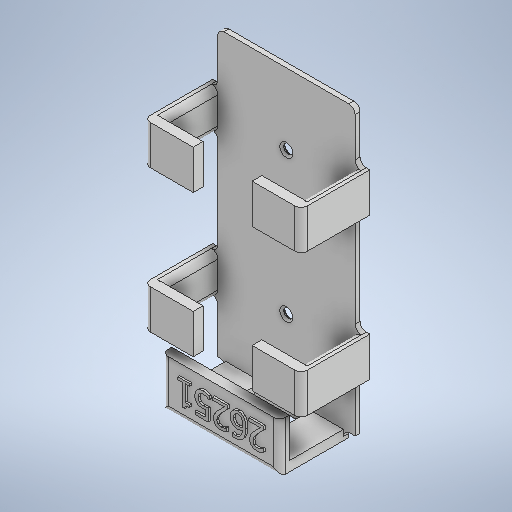
# Autodesk Inventor part: ChonkyPowerBankHolder
Saved by Autodesk Inventor 2025 (Build 290162010, 162A)
## iProperties
Created: 2024-11-16
Part Number: ChonkyPowerBankHolder
Material: Generic
Document SubType Name: Modeling
Designer: ishaa
Density: 1 g/cm^3
Appearance: Default
Author: ishaa
## iProperties of the stored document ChonkyPowerBankHolder_3DPrint.ipt
Created: 2024-12-01
Part Number: ChonkyPowerBankHolder_3DPrint
Material: Generic
Document SubType Name: Modeling
Designer: dcfam
Density: 1 g/cm^3
Appearance: Default
Author: dcfam
Autodesk Inventor part; units mm, degrees
ref_plane "YZ Plane" through (0, 0, 0) normal (1, 0, 0) x (0, 1, 0)
ref_plane "XZ Plane" through (0, 0, 0) normal (0, 1, 0) x (-1, 0, 0)
ref_plane "XY Plane" through (0, 0, 0) normal (0, 0, 1) x (1, 0, 0)
sketch "Sketch1" plane through (0, 0, 0) normal (0, 0, 1) x (1, 0, 0)
  line L0 (-35, -72.5) -> (35, -72.5)
  line L1 (35, -72.5) -> (35, 72.5)
  line L2 (35, 72.5) -> (-35, 72.5)
  line L3 (-35, 72.5) -> (-35, -72.5)
  line L4 (-35, -72.5) -> (35, 72.5) construction
  line L5 (35, -72.5) -> (-35, 72.5) construction
  point P0 (0, 0)
  dimension "d0" = 70
  dimension "d1" = 145
  constraints: 12 end point, 2 midpoint, 2 parallel, 1 horizontal, 1 perpendicular
  measures "d0" distance of L2.end L1.end
  measures "d1" distance of L1.end L0.end
extrude "Extrusion1" add sketch "Sketch1" along normal blind 2.5
sketch "Sketch2" plane through (0, 0, 0) normal (0, 0, -1) x (-1, 0, 0)
  line L0 (-35, 72.5) -> (35, 72.5) construction
  line L1 (0, 72.5) -> (0, -72.5) construction
  line L2 (35, -72.5) -> (-35, -72.5) construction
  line L3 (35, 0) -> (-35, 0) construction
  line L4 (-35, -72.5) -> (-35, 72.5) construction
  line L5 (-35, 0) -> (-35, -72.5) construction
  line L6 (-35, -36.25) -> (35, -36.25) construction
  line L7 (35, 72.5) -> (35, -72.5) construction
  line L8 (-35, -72.5) -> (-35, 72.5) construction
  line L9 (-35, 72.5) -> (35, 72.5) construction
  line L10 (35, 72.5) -> (35, -72.5) construction
  line L11 (35, -72.5) -> (-35, -72.5) construction
  line L12 (-35, 72.5) -> (-35, 0) construction
  line L13 (-35, 36.25) -> (35, 36.25) construction
  line L14 (-35, 46.25) -> (-40, 46.25)
  line L15 (-40, 46.25) -> (-40, 26.25)
  line L16 (-40, 26.25) -> (-35, 26.25)
  line L17 (-35, 26.25) -> (-35, 46.25)
  line L18 (-35, 36.25) -> (-23.1595, 36.25) construction
  line L19 (35, 46.25) -> (40, 46.25)
  line L20 (40, 46.25) -> (40, 26.25)
  line L21 (40, 26.25) -> (35, 26.25)
  line L22 (35, 26.25) -> (35, 46.25)
  line L23 (-35, -46.25) -> (-40, -46.25)
  line L24 (-40, -46.25) -> (-40, -26.25)
  line L25 (-40, -26.25) -> (-35, -26.25)
  line L26 (-35, -26.25) -> (-35, -46.25)
  line L27 (40, -26.25) -> (35, -26.25)
  line L28 (40, -46.25) -> (40, -26.25)
  line L29 (35, -46.25) -> (40, -46.25)
  line L30 (35, -26.25) -> (35, -46.25)
  line L31 (-29.0797, -72.5) -> (30.9203, -72.5)
  line L32 (30.9203, -72.5) -> (30.9203, -77.5)
  line L33 (30.9203, -77.5) -> (-29.0797, -77.5)
  line L34 (-29.0797, -77.5) -> (-29.0797, -72.5)
  point P0 (0, 0)
  dimension "d4" = 5
  dimension "d5" = 20
  dimension "d6" = 60
  dimension "d7" = 5
  constraints: 54 end point, 12 symmetric about line, 6 midpoint, 4 parallel, 4 perpendicular, 4 point on line, 3 collinear, 3 horizontal
  measures "d4" distance of L16.end L15.end
  measures "d5" distance of L15.end L14.end
  measures "d6" distance of L32.end L33.end
  measures "d7" distance of L31.end L32.end
extrude "Extrusion2" add sketch "Sketch2" against normal blind 35
sketch "Sketch3" plane through (-30.9203, -72.5, 2.5) normal (0, 1, 0) x (1, 0, 0)
  line L0 (0, 0) -> (60, 0) projected
  line L1 (0, 0) -> (0, -32.5) projected
  line L2 (60, -32.5) -> (0, -32.5) projected
  line L3 (60, 0) -> (60, -32.5) projected
  line L4 (60, -32.5) -> (0, -32.5)
  line L5 (0, -32.5) -> (0, -27.5)
  line L6 (0, -27.5) -> (60, -27.5)
  line L7 (60, -27.5) -> (60, -32.5)
  point P0 (30.9203, 2.5)
  dimension "d10" = 5
  constraints: 8 end point, 2 parallel, 1 horizontal, 1 perpendicular, 1 point on line
  measures "d10" distance of L4.end L5.end
sketch "Sketch4" plane through (35, 26.25, 2.5) normal (-1, 0, 0) x (0, 0, 1)
  line L0 (0, 0) -> (0, 20) projected
  line L1 (0, 0) -> (32.5, 0) projected
  line L2 (32.5, 20) -> (32.5, 0) projected
  line L3 (0, 20) -> (32.5, 20) projected
  line L4 (0, -72.5) -> (0, -52.5) projected
  line L5 (0, -72.5) -> (32.5, -72.5) projected
  line L6 (32.5, -52.5) -> (32.5, -72.5) projected
  line L7 (0, -52.5) -> (32.5, -52.5) projected
  line L8 (32.5, 20) -> (27.5, 20)
  line L9 (27.5, 20) -> (27.5, 0)
  line L10 (27.5, 0) -> (32.5, 0)
  line L11 (32.5, 0) -> (32.5, 20)
  line L12 (0, -52.5) -> (0, 0) projected
  line L13 (0, -26.25) -> (53.9685, -26.25) construction
  line L14 (0, -52.5) -> (32.5, -52.5)
  line L15 (32.5, -72.5) -> (32.5, -52.5)
  line L16 (0, -72.5) -> (32.5, -72.5)
  line L17 (27.5, -72.5) -> (27.5, -52.5)
  point P0 (-2.5, -26.25)
  dimension "d11" = 5
  constraints: 18 end point, 3 symmetric about line, 2 horizontal, 2 parallel, 2 point on line, 1 midpoint, 1 perpendicular
  measures "d11" distance of L10.end L9.end
sketch "Sketch5" plane through (-35, -46.25, 2.5) normal (1, 0, 0) x (0, 0, -1)
  line L0 (0, 0) -> (-32.5, 0) projected
  line L1 (2.5, 20) -> (-32.5, 20) projected
  line L2 (-32.5, 0) -> (-27.5, 0)
  line L3 (-27.5, 0) -> (-27.5, 20)
  line L4 (-27.5, 20) -> (-32.5, 20)
  line L5 (-32.5, 20) -> (-32.5, 0)
  line L6 (0, 72.5) -> (0, 20) construction
  line L7 (0, 46.25) -> (-51.5825, 46.25) construction
  line L8 (-32.5, 92.5) -> (-27.5, 92.5)
  line L9 (-27.5, 92.5) -> (-27.5, 72.5)
  line L10 (-27.5, 72.5) -> (-32.5, 72.5)
  line L11 (-32.5, 72.5) -> (-32.5, 92.5)
  point P0 (2.5, 46.25)
  dimension "d12" = 5
  constraints: 18 end point, 4 symmetric about line, 2 horizontal, 2 parallel, 1 midpoint, 1 perpendicular, 1 point on line
  measures "d12" distance of L4.end L3.end
extrude "Extrusion3" add sketch "Sketch3" along normal blind 20 contours L6 L3 L2 L1
extrude "Extrusion4" add sketch "Sketch5" along normal blind 20
extrude "Extrusion5" add sketch "Sketch4" along normal blind 20 contours L9 L3 L2 L1 | L17 L7 L6 L5
sketch "Sketch6" plane through (0, 0, 2.5) normal (0, 0, 1) x (1, 0, 0)
  line L0 (-30.9203, -77.5) -> (29.0797, -77.5) construction
  line L1 (0, -77.5) -> (0, 72.5) construction
  line L2 (35, 72.5) -> (-35, 72.5) construction
  line L3 (-40, -26.25) -> (-40, -46.25) construction
  line L4 (-40, -46.25) -> (-15, -46.25) construction
  line L5 (-15, -26.25) -> (-15, -46.25) construction
  line L6 (-40, -26.25) -> (-15, -26.25) construction
  line L7 (-15, -26.25) -> (-15, -46.25) construction
  line L8 (-15, -36.25) -> (15, -36.25) construction
  line L9 (15, -46.25) -> (15, -26.25) construction
  circle A0 centre (0, -36.25) radius 2.35
  line L10 (-35, 26.25) -> (-35, -26.25) construction
  line L11 (-35, 0) -> (35, 0) construction
  circle A1 centre (0, 36.25) radius 2.35
  point P0 (0, 0)
  dimension "d19" = 4.7
  constraints: 6 end point, 5 midpoint, 2 centre point, 1 horizontal, 1 point on line, 1 symmetric about line, 1 other
  measures "d19" diameter of A0
extrude "Extrusion6" cut sketch "Sketch6" against normal blind 20
chamfer "Chamfer1" distance 1 angle 45 4 edges at (-2.35, -36.25, 2.5) (-2.35, 36.25, 2.5) (-2.35, -36.25, 0) (-2.35, 36.25, 0)
fillet "Fillet1" radius 3.175 10 edges at (35, -46.25, 1.25) (35, -26.25, 1.25) (35, 46.25, 1.25) (35, 26.25, 1.25) (29.0797, -72.5, 1.25) (-30.9203, -72.5, 1.25) (-35, -46.25, 1.25) (-35, -26.25, 1.25) (-35, 26.25, 1.25) (-35, 46.25, 1.25)
fillet "Fillet2" radius 3.175 2 edges at (-35, 72.5, 1.25) (35, 72.5, 1.25)
fillet "Fillet3" radius 3.175 4 edges at (-40, -36.25, 35) (-40, 36.25, 35) (40, -36.25, 35) (40, 36.25, 35)
fillet "Fillet4" radius 3.175 3 edges at (-0.9203, -77.5, 35) (-30.9203, -65, 35) (29.0797, -65, 35)
fillet "Fillet5" radius 3.175 8 edges at (-35, 46.25, 16.25) (35, 46.25, 16.25) (-35, -26.25, 16.25) (35, -26.25, 16.25) (-35, 26.25, 16.25) (35, 26.25, 16.25) (35, -46.25, 16.25) (-35, -46.25, 16.25)
sketch "Sketch7" plane through (0, 0, 35) normal (0, 0, 1) x (1, 0, 0)
  line L0 (22.7543, -70.5434) -> (-153.14, -70.5434) construction
  line L1 (-153.14, -70.5434) -> (-153.14, -5.5157) construction
  line L2 (-153.14, -5.5157) -> (22.7543, -5.5157) construction
  line L3 (22.7543, -5.5157) -> (22.7543, -70.5434) construction
  line L4 (14.303, -58.0303) -> (21.8606, -58.0303)
  line L5 (21.8606, -58.0303) -> (21.8606, -59.7682)
  spline S0 degree 2 poles (21.8606, -59.7682) (21.0462, -60.5329) (19.5963, -61.953) (18.9011, -62.7177) knots 0 0 0 1 2 2 2
  spline S1 degree 2 poles (18.9011, -62.7177) (17.5008, -64.257) (16.4779, -66.1042) (16.4779, -67.0874) knots 0 0 0 1 2 2 2
  spline S2 degree 2 poles (16.4779, -67.0874) (16.4779, -67.6038) (16.7957, -68.3784) (17.0837, -68.6267) knots 0 0 0 1 2 2 2
  spline S3 degree 2 poles (17.0837, -68.6267) (17.3717, -68.875) (18.1265, -69.1232) (18.5833, -69.1232) knots 0 0 0 1 2 2 2
  spline S4 degree 2 poles (18.5833, -69.1232) (19.0203, -69.1232) (19.9141, -68.9047) (20.3212, -68.7359) knots 0 0 0 1 2 2 2
  spline S5 degree 2 poles (20.3212, -68.7359) (20.6688, -68.5969) (21.3143, -68.1996) (21.513, -68.0606) knots 0 0 0 1 2 2 2
  line L6 (21.513, -68.0606) -> (21.6023, -68.0606)
  line L7 (21.6023, -68.0606) -> (21.6023, -69.8085)
  spline S6 degree 2 poles (21.6023, -69.8085) (21.0959, -70.0567) (19.2785, -70.5434) (18.4641, -70.5434) knots 0 0 0 1 2 2 2
  spline S7 degree 2 poles (18.4641, -70.5434) (16.7461, -70.5434) (14.8095, -68.726) (14.8095, -67.1767) knots 0 0 0 1 2 2 2
  spline S8 degree 2 poles (14.8095, -67.1767) (14.8095, -66.4518) (15.1472, -65.2402) (15.4451, -64.7238) knots 0 0 0 1 2 2 2
  spline S9 degree 2 poles (15.4451, -64.7238) (15.743, -64.1875) (16.607, -63.1348) (17.0837, -62.6283) knots 0 0 0 1 2 2 2
  spline S10 degree 2 poles (17.0837, -62.6283) (17.8583, -61.7842) (19.7552, -59.9768) (20.3212, -59.4504) knots 0 0 0 1 2 2 2
  line L8 (20.3212, -59.4504) -> (14.303, -59.4504)
  line L9 (14.303, -59.4504) -> (14.303, -58.0303)
  spline S11 degree 2 poles (4.9182, -62.0027) (4.9182, -61.0592) (5.5439, -59.4603) (6.0702, -58.9241) knots 0 0 0 1 2 2 2
  spline S12 degree 2 poles (6.0702, -58.9241) (6.6164, -58.358) (7.9869, -57.7721) (8.8112, -57.7721) knots 0 0 0 1 2 2 2
  spline S13 degree 2 poles (8.8112, -57.7721) (9.6355, -57.7721) (10.996, -58.3282) (11.5124, -58.8843) knots 0 0 0 1 2 2 2
  spline S14 degree 2 poles (11.5124, -58.8843) (12.148, -59.5497) (12.863, -61.7842) (12.863, -63.4129) knots 0 0 0 1 2 2 2
  spline S15 degree 2 poles (12.863, -63.4129) (12.863, -65.0118) (12.2076, -67.5839) (11.5223, -68.5373) knots 0 0 0 1 2 2 2
  spline S16 degree 2 poles (11.5223, -68.5373) (10.857, -69.4708) (8.7516, -70.5136) (7.3712, -70.5136) knots 0 0 0 1 2 2 2
  spline S17 degree 2 poles (7.3712, -70.5136) (6.964, -70.5136) (6.249, -70.4341) (5.9808, -70.3447) knots 0 0 0 1 2 2 2
  line L10 (5.9808, -70.3447) -> (5.9808, -68.7657)
  line L11 (5.9808, -68.7657) -> (6.0504, -68.7657)
  spline S18 degree 2 poles (6.0504, -68.7657) (6.2788, -68.8849) (7.113, -69.0934) (7.5897, -69.0934) knots 0 0 0 1 2 2 2
  spline S19 degree 2 poles (7.5897, -69.0934) (9.119, -69.0934) (10.996, -67.0278) (11.1748, -65.0019) knots 0 0 0 1 2 2 2
  spline S20 degree 2 poles (11.1748, -65.0019) (10.5888, -65.409) (9.3574, -65.8559) (8.6225, -65.8559) knots 0 0 0 1 2 2 2
  spline S21 degree 2 poles (8.6225, -65.8559) (7.9075, -65.8559) (6.8349, -65.5679) (6.249, -65.131) knots 0 0 0 1 2 2 2
  spline S22 degree 2 poles (6.249, -65.131) (5.5737, -64.6245) (4.9182, -63.0554) (4.9182, -62.0027) knots 0 0 0 1 2 2 2
  spline S23 degree 2 poles (6.5866, -61.9332) (6.5866, -62.6879) (6.9839, -63.7108) (7.4208, -64.0683) knots 0 0 0 1 2 2 2
  spline S24 degree 2 poles (7.4208, -64.0683) (7.7486, -64.3265) (8.5629, -64.4954) (8.9899, -64.4954) knots 0 0 0 1 2 2 2
  spline S25 degree 2 poles (8.9899, -64.4954) (9.5659, -64.4954) (10.6484, -64.1478) (11.1748, -63.8201) knots 0 0 0 1 2 2 2
  spline S26 degree 2 poles (11.1748, -63.8201) (11.1847, -63.6413) (11.2046, -63.3036) (11.2046, -63.0454) knots 0 0 0 1 2 2 2
  spline S27 degree 2 poles (11.2046, -63.0454) (11.2046, -61.7743) (10.708, -60.2151) (10.3306, -59.8079) knots 0 0 0 1 2 2 2
  spline S28 degree 2 poles (10.3306, -59.8079) (9.983, -59.4206) (9.2283, -59.1128) (8.8012, -59.1128) knots 0 0 0 1 2 2 2
  spline S29 degree 2 poles (8.8012, -59.1128) (7.8081, -59.1128) (6.5866, -60.523) (6.5866, -61.9332) knots 0 0 0 1 2 2 2
  line L12 (-4.0892, -58.0303) -> (3.4683, -58.0303)
  line L13 (3.4683, -58.0303) -> (3.4683, -59.7682)
  spline S30 degree 2 poles (3.4683, -59.7682) (2.6539, -60.5329) (1.204, -61.953) (0.5088, -62.7177) knots 0 0 0 1 2 2 2
  spline S31 degree 2 poles (0.5088, -62.7177) (-0.8914, -64.257) (-1.9143, -66.1042) (-1.9143, -67.0874) knots 0 0 0 1 2 2 2
  spline S32 degree 2 poles (-1.9143, -67.0874) (-1.9143, -67.6038) (-1.5965, -68.3784) (-1.3085, -68.6267) knots 0 0 0 1 2 2 2
  spline S33 degree 2 poles (-1.3085, -68.6267) (-1.0205, -68.875) (-0.2658, -69.1232) (0.191, -69.1232) knots 0 0 0 1 2 2 2
  spline S34 degree 2 poles (0.191, -69.1232) (0.628, -69.1232) (1.5218, -68.9047) (1.929, -68.7359) knots 0 0 0 1 2 2 2
  spline S35 degree 2 poles (1.929, -68.7359) (2.2766, -68.5969) (2.9221, -68.1996) (3.1207, -68.0606) knots 0 0 0 1 2 2 2
  line L14 (3.1207, -68.0606) -> (3.2101, -68.0606)
  line L15 (3.2101, -68.0606) -> (3.2101, -69.8085)
  spline S36 degree 2 poles (3.2101, -69.8085) (2.7036, -70.0567) (0.8862, -70.5434) (0.0719, -70.5434) knots 0 0 0 1 2 2 2
  spline S37 degree 2 poles (0.0719, -70.5434) (-1.6462, -70.5434) (-3.5827, -68.726) (-3.5827, -67.1767) knots 0 0 0 1 2 2 2
  spline S38 degree 2 poles (-3.5827, -67.1767) (-3.5827, -66.4518) (-3.2451, -65.2402) (-2.9472, -64.7238) knots 0 0 0 1 2 2 2
  spline S39 degree 2 poles (-2.9472, -64.7238) (-2.6492, -64.1875) (-1.7852, -63.1348) (-1.3085, -62.6283) knots 0 0 0 1 2 2 2
  spline S40 degree 2 poles (-1.3085, -62.6283) (-0.5339, -61.7842) (1.3629, -59.9768) (1.929, -59.4504) knots 0 0 0 1 2 2 2
  line L16 (1.929, -59.4504) -> (-4.0892, -59.4504)
  line L17 (-4.0892, -59.4504) -> (-4.0892, -58.0303)
  spline S41 degree 2 poles (-13.1563, -61.9232) (-13.1563, -61.0394) (-12.5902, -59.5299) (-12.0738, -58.9737) knots 0 0 0 1 2 2 2
  spline S42 degree 2 poles (-12.0738, -58.9737) (-11.5574, -58.4176) (-10.0181, -57.7721) (-9.0647, -57.7721) knots 0 0 0 1 2 2 2
  spline S43 degree 2 poles (-9.0647, -57.7721) (-8.1907, -57.7721) (-6.4826, -58.1594) (-5.857, -58.4672) knots 0 0 0 1 2 2 2
  line L18 (-5.857, -58.4672) -> (-5.857, -60.2052)
  line L19 (-5.857, -60.2052) -> (-5.9761, -60.2052)
  spline S44 degree 2 poles (-5.9761, -60.2052) (-6.1648, -60.0661) (-6.8699, -59.7086) (-7.297, -59.5497) knots 0 0 0 1 2 2 2
  spline S45 degree 2 poles (-7.297, -59.5497) (-7.7836, -59.3809) (-8.588, -59.1922) (-9.0945, -59.1922) knots 0 0 0 1 2 2 2
  spline S46 degree 2 poles (-9.0945, -59.1922) (-9.591, -59.1922) (-10.5245, -59.5497) (-10.8622, -59.937) knots 0 0 0 1 2 2 2
  spline S47 degree 2 poles (-10.8622, -59.937) (-11.1701, -60.3045) (-11.4878, -61.2777) (-11.4878, -61.9332) knots 0 0 0 1 2 2 2
  spline S48 degree 2 poles (-11.4878, -61.9332) (-11.4878, -62.5886) (-11.1303, -63.4228) (-10.7927, -63.7009) knots 0 0 0 1 2 2 2
  spline S49 degree 2 poles (-10.7927, -63.7009) (-10.4451, -64.0087) (-9.4123, -64.267) (-8.7866, -64.267) knots 0 0 0 1 2 2 2
  spline S50 degree 2 poles (-8.7866, -64.267) (-8.1113, -64.267) (-6.7706, -64.0584) (-6.3634, -63.969) knots 0 0 0 1 2 2 2
  line L20 (-6.3634, -63.969) -> (-6.3634, -70.2852)
  line L21 (-6.3634, -70.2852) -> (-13.0867, -70.2852)
  line L22 (-13.0867, -70.2852) -> (-13.0867, -68.8452)
  line L23 (-13.0867, -68.8452) -> (-7.9425, -68.8452)
  line L24 (-7.9425, -68.8452) -> (-7.9425, -65.5779)
  spline S51 degree 2 poles (-7.9425, -65.5779) (-8.2404, -65.6176) (-8.8164, -65.6474) (-9.0547, -65.6474) knots 0 0 0 1 2 2 2
  spline S52 degree 2 poles (-9.0547, -65.6474) (-9.9982, -65.6474) (-11.2992, -65.3395) (-11.895, -64.8827) knots 0 0 0 1 2 2 2
  spline S53 degree 2 poles (-11.895, -64.8827) (-12.5008, -64.4259) (-13.1563, -63.0355) (-13.1563, -61.9232) knots 0 0 0 1 2 2 2
  line L25 (-21.8658, -58.0303) -> (-15.8873, -58.0303)
  line L26 (-15.8873, -58.0303) -> (-15.8873, -59.2816)
  line L27 (-15.8873, -59.2816) -> (-18.1118, -59.2816)
  line L28 (-18.1118, -59.2816) -> (-18.1118, -67.4945)
  line L29 (-18.1118, -67.4945) -> (-15.8873, -67.4945)
  line L30 (-15.8873, -67.4945) -> (-15.8873, -68.6167)
  spline S54 degree 2 poles (-15.8873, -68.6167) (-17.1485, -68.6167) (-18.3403, -69.3318) (-18.4197, -70.3249) knots 0 0 0 1 2 2 2
  line L31 (-18.4197, -70.3249) -> (-19.6909, -70.3249)
  line L32 (-19.6909, -70.3249) -> (-19.6909, -59.2816)
  line L33 (-19.6909, -59.2816) -> (-21.8658, -59.2816)
  line L34 (-21.8658, -59.2816) -> (-21.8658, -58.0303)
  point P0 (0, 0)
  constraints: 2 other
emboss "Emboss1" sketch "Sketch7" operation add depth 1 direction (0, 0, -1)
sketch "Sketch8" plane through (-30.9203, -77.5, 0) normal (0, -1, 0) x (1, 0, 0)
  line L0 (0, 31.825) -> (60, 31.825) construction
  line L1 (30.9203, 31.825) -> (30.9203, 0) construction
  line L2 (0, 0) -> (0, 31.825) construction
  line L3 (0, 15.9125) -> (60, 16.25) construction
  line L4 (60, 2.5) -> (60, 30) construction
  line L5 (18.4203, 6.0864) -> (43.4203, 6.0864)
  line L6 (43.4203, 6.0864) -> (43.4203, 26.0864)
  line L7 (43.4203, 26.0864) -> (18.4203, 26.0864)
  line L8 (18.4203, 26.0864) -> (18.4203, 6.0864)
  line L9 (18.4203, 6.0864) -> (43.4203, 26.0864) construction
  line L10 (43.4203, 6.0864) -> (18.4203, 26.0864) construction
  point P0 (30.9203, 16.0864)
  dimension "d32" = 25
  dimension "d33" = 20
  constraints: 16 end point, 4 midpoint, 3 point on line, 2 parallel, 1 horizontal, 1 perpendicular, 1 vertical
  measures "d32" distance of L7.end L6.end
  measures "d33" distance of L6.end L5.end
extrude "Extrusion7" cut sketch "Sketch8" against normal blind 25.4
sketch "Sketch9" plane through (-30.9203, -77.5, 0) normal (0, -1, 0) x (1, 0, 0)
  line L0 (20.1191, 30.5811) -> (41.7214, 30.5811) construction
  line L1 (41.7214, 30.5811) -> (41.7214, 26.6961) construction
  line L2 (41.7214, 26.6961) -> (20.1191, 26.6961) construction
  line L3 (20.1191, 26.6961) -> (20.1191, 30.5811) construction
  line L4 (30.9203, 26.6961) -> (30.9203, 23.2384) construction
  line L5 (43.4203, 26.0864) -> (18.4203, 26.0864) projected
  spline S0 degree 2 poles (22.3544, 29.6079) (22.3544, 29.4103) (22.2136, 29.0546) (22.0877, 28.9311) knots 0 0 0 1 2 2 2
  spline S1 degree 2 poles (22.0877, 28.9311) (21.9296, 28.7755) (21.5023, 28.615) (21.1762, 28.615) knots 0 0 0 1 2 2 2
  line L6 (21.1762, 28.615) -> (20.8329, 28.615)
  line L7 (20.8329, 28.615) -> (20.8329, 27.4788)
  line L8 (20.8329, 27.4788) -> (20.4278, 27.4788)
  line L9 (20.4278, 27.4788) -> (20.4278, 30.5268)
  line L10 (20.4278, 30.5268) -> (21.1935, 30.5268)
  spline S2 degree 2 poles (21.1935, 30.5268) (21.4652, 30.5268) (21.8456, 30.4378) (21.9913, 30.3366) knots 0 0 0 1 2 2 2
  spline S3 degree 2 poles (21.9913, 30.3366) (22.1618, 30.2205) (22.3544, 29.8623) (22.3544, 29.6079) knots 0 0 0 1 2 2 2
  spline S4 degree 2 poles (21.9321, 29.5956) (21.9321, 29.7536) (21.8234, 29.9858) (21.7122, 30.0599) knots 0 0 0 1 2 2 2
  spline S5 degree 2 poles (21.7122, 30.0599) (21.6159, 30.1241) (21.359, 30.176) (21.1688, 30.176) knots 0 0 0 1 2 2 2
  line L11 (21.1688, 30.176) -> (20.8329, 30.176)
  line L12 (20.8329, 30.176) -> (20.8329, 28.9608)
  line L13 (20.8329, 28.9608) -> (21.1095, 28.9608)
  spline S6 degree 2 poles (21.1095, 28.9608) (21.3565, 28.9608) (21.6603, 29.0398) (21.7592, 29.1435) knots 0 0 0 1 2 2 2
  spline S7 degree 2 poles (21.7592, 29.1435) (21.8505, 29.2349) (21.9321, 29.4498) (21.9321, 29.5956) knots 0 0 0 1 2 2 2
  spline S8 degree 2 poles (23.8043, 27.4145) (23.5351, 27.4145) (23.1349, 27.5553) (22.9942, 27.6961) knots 0 0 0 1 2 2 2
  spline S9 degree 2 poles (22.9942, 27.6961) (22.8336, 27.8542) (22.7027, 28.2988) (22.7027, 28.6248) knots 0 0 0 1 2 2 2
  line L14 (22.7027, 28.6248) -> (22.7027, 30.5268)
  line L15 (22.7027, 30.5268) -> (23.1078, 30.5268)
  line L16 (23.1078, 30.5268) -> (23.1078, 28.6248)
  spline S10 degree 2 poles (23.1078, 28.6248) (23.1078, 28.4124) (23.1621, 28.1259) (23.2387, 28.0098) knots 0 0 0 1 2 2 2
  spline S11 degree 2 poles (23.2387, 28.0098) (23.3202, 27.8863) (23.6018, 27.7603) (23.8043, 27.7603) knots 0 0 0 1 2 2 2
  spline S12 degree 2 poles (23.8043, 27.7603) (23.9945, 27.7603) (24.2909, 27.8863) (24.3724, 28.0098) knots 0 0 0 1 2 2 2
  spline S13 degree 2 poles (24.3724, 28.0098) (24.449, 28.1259) (24.5033, 28.41) (24.5033, 28.615) knots 0 0 0 1 2 2 2
  line L17 (24.5033, 28.615) -> (24.5033, 30.5268)
  line L18 (24.5033, 30.5268) -> (24.9084, 30.5268)
  line L19 (24.9084, 30.5268) -> (24.9084, 28.6248)
  spline S14 degree 2 poles (24.9084, 28.6248) (24.9084, 28.3062) (24.78, 27.8517) (24.617, 27.6961) knots 0 0 0 1 2 2 2
  spline S15 degree 2 poles (24.617, 27.6961) (24.4712, 27.5529) (24.0859, 27.4145) (23.8043, 27.4145) knots 0 0 0 1 2 2 2
  spline S16 degree 2 poles (26.3386, 27.4244) (26.0076, 27.4244) (25.5432, 27.5627) (25.3382, 27.6615) knots 0 0 0 1 2 2 2
  line L20 (25.3382, 27.6615) -> (25.3382, 28.1704)
  line L21 (25.3382, 28.1704) -> (25.3678, 28.1704)
  spline S17 degree 2 poles (25.3678, 28.1704) (25.5679, 27.9826) (26.0743, 27.7752) (26.3089, 27.7752) knots 0 0 0 1 2 2 2
  spline S18 degree 2 poles (26.3089, 27.7752) (26.6448, 27.7752) (26.9882, 28.0543) (26.9882, 28.284) knots 0 0 0 1 2 2 2
  spline S19 degree 2 poles (26.9882, 28.284) (26.9882, 28.4668) (26.8079, 28.694) (26.6127, 28.7508) knots 0 0 0 1 2 2 2
  spline S20 degree 2 poles (26.6127, 28.7508) (26.4719, 28.7903) (26.2373, 28.8447) (26.0619, 28.8891) knots 0 0 0 1 2 2 2
  spline S21 degree 2 poles (26.0619, 28.8891) (25.9038, 28.9311) (25.6544, 29.0571) (25.558, 29.1584) knots 0 0 0 1 2 2 2
  spline S22 degree 2 poles (25.558, 29.1584) (25.4642, 29.2596) (25.3604, 29.5313) (25.3604, 29.7092) knots 0 0 0 1 2 2 2
  spline S23 degree 2 poles (25.3604, 29.7092) (25.3604, 30.0797) (25.9384, 30.5811) (26.3855, 30.5811) knots 0 0 0 1 2 2 2
  spline S24 degree 2 poles (26.3855, 30.5811) (26.6424, 30.5811) (27.0969, 30.4798) (27.292, 30.3835) knots 0 0 0 1 2 2 2
  line L22 (27.292, 30.3835) -> (27.292, 29.8994)
  line L23 (27.292, 29.8994) -> (27.2623, 29.8994)
  spline S25 degree 2 poles (27.2623, 29.8994) (27.1166, 30.0328) (26.6621, 30.2304) (26.4127, 30.2304) knots 0 0 0 1 2 2 2
  spline S26 degree 2 poles (26.4127, 30.2304) (26.1311, 30.2304) (25.7828, 29.9661) (25.7828, 29.7512) knots 0 0 0 1 2 2 2
  spline S27 degree 2 poles (25.7828, 29.7512) (25.7828, 29.5585) (25.9878, 29.3288) (26.1805, 29.2769) knots 0 0 0 1 2 2 2
  spline S28 degree 2 poles (26.1805, 29.2769) (26.3089, 29.2423) (26.6819, 29.1534) (26.8054, 29.1164) knots 0 0 0 1 2 2 2
  spline S29 degree 2 poles (26.8054, 29.1164) (27.1191, 29.02) (27.4105, 28.6323) (27.4105, 28.3482) knots 0 0 0 1 2 2 2
  spline S30 degree 2 poles (27.4105, 28.3482) (27.4105, 28.1679) (27.2648, 27.8221) (27.1339, 27.7011) knots 0 0 0 1 2 2 2
  spline S31 degree 2 poles (27.1339, 27.7011) (26.9882, 27.5677) (26.6177, 27.4244) (26.3386, 27.4244) knots 0 0 0 1 2 2 2
  line L24 (30.0362, 27.4788) -> (29.6311, 27.4788)
  line L25 (29.6311, 27.4788) -> (29.6311, 28.9706)
  line L26 (29.6311, 28.9706) -> (28.2281, 28.9706)
  line L27 (28.2281, 28.9706) -> (28.2281, 27.4788)
  line L28 (28.2281, 27.4788) -> (27.823, 27.4788)
  line L29 (27.823, 27.4788) -> (27.823, 30.5268)
  line L30 (27.823, 30.5268) -> (28.2281, 30.5268)
  line L31 (28.2281, 30.5268) -> (28.2281, 29.3313)
  line L32 (28.2281, 29.3313) -> (29.6311, 29.3313)
  line L33 (29.6311, 29.3313) -> (29.6311, 30.5268)
  line L34 (29.6311, 30.5268) -> (30.0362, 30.5268)
  line L35 (30.0362, 30.5268) -> (30.0362, 27.4788)
  line L36 (34.1759, 27.4788) -> (33.7708, 27.4788)
  line L37 (33.7708, 27.4788) -> (33.7708, 28.9706)
  line L38 (33.7708, 28.9706) -> (32.3679, 28.9706)
  line L39 (32.3679, 28.9706) -> (32.3679, 27.4788)
  line L40 (32.3679, 27.4788) -> (31.9628, 27.4788)
  line L41 (31.9628, 27.4788) -> (31.9628, 30.5268)
  line L42 (31.9628, 30.5268) -> (32.3679, 30.5268)
  line L43 (32.3679, 30.5268) -> (32.3679, 29.3313)
  line L44 (32.3679, 29.3313) -> (33.7708, 29.3313)
  line L45 (33.7708, 29.3313) -> (33.7708, 30.5268)
  line L46 (33.7708, 30.5268) -> (34.1759, 30.5268)
  line L47 (34.1759, 30.5268) -> (34.1759, 27.4788)
  line L48 (34.7934, 27.4788) -> (34.7934, 30.5268)
  line L49 (34.7934, 30.5268) -> (36.7003, 30.5268)
  line L50 (36.7003, 30.5268) -> (36.7003, 30.1661)
  line L51 (36.7003, 30.1661) -> (35.1985, 30.1661)
  line L52 (35.1985, 30.1661) -> (35.1985, 29.3313)
  line L53 (35.1985, 29.3313) -> (36.599, 29.3313)
  line L54 (36.599, 29.3313) -> (36.599, 28.9706)
  line L55 (36.599, 28.9706) -> (35.1985, 28.9706)
  line L56 (35.1985, 28.9706) -> (35.1985, 27.8394)
  line L57 (35.1985, 27.8394) -> (36.7003, 27.8394)
  line L58 (36.7003, 27.8394) -> (36.7003, 27.4788)
  line L59 (36.7003, 27.4788) -> (34.7934, 27.4788)
  line L60 (39.5037, 27.4788) -> (38.9776, 27.4788)
  line L61 (38.9776, 27.4788) -> (38.0143, 28.6915)
  line L62 (38.0143, 28.6915) -> (37.55, 28.6915)
  line L63 (37.55, 28.6915) -> (37.55, 27.4788)
  line L64 (37.55, 27.4788) -> (37.1449, 27.4788)
  line L65 (37.1449, 27.4788) -> (37.1449, 30.5268)
  line L66 (37.1449, 30.5268) -> (37.9303, 30.5268)
  spline S32 degree 2 poles (37.9303, 30.5268) (38.1922, 30.5268) (38.5454, 30.4699) (38.7059, 30.3662) knots 0 0 0 1 2 2 2
  spline S33 degree 2 poles (38.7059, 30.3662) (38.8665, 30.2625) (39.0517, 29.9389) (39.0517, 29.6993) knots 0 0 0 1 2 2 2
  spline S34 degree 2 poles (39.0517, 29.6993) (39.0517, 29.3658) (38.7109, 28.9138) (38.4194, 28.8052) knots 0 0 0 1 2 2 2
  line L67 (38.4194, 28.8052) -> (39.5037, 27.4788)
  spline S35 degree 2 poles (38.6294, 29.6672) (38.6294, 29.8006) (38.5355, 30.0056) (38.4367, 30.0723) knots 0 0 0 1 2 2 2
  spline S36 degree 2 poles (38.4367, 30.0723) (38.3502, 30.1291) (38.1205, 30.176) (37.9526, 30.176) knots 0 0 0 1 2 2 2
  line L68 (37.9526, 30.176) -> (37.55, 30.176)
  line L69 (37.55, 30.176) -> (37.55, 29.0299)
  line L70 (37.55, 29.0299) -> (37.9056, 29.0299)
  spline S37 degree 2 poles (37.9056, 29.0299) (38.081, 29.0299) (38.3601, 29.0917) (38.4565, 29.188) knots 0 0 0 1 2 2 2
  spline S38 degree 2 poles (38.4565, 29.188) (38.5454, 29.272) (38.6294, 29.5091) (38.6294, 29.6672) knots 0 0 0 1 2 2 2
  line L71 (39.7458, 27.4788) -> (39.7458, 30.5268)
  line L72 (39.7458, 30.5268) -> (41.6527, 30.5268)
  line L73 (41.6527, 30.5268) -> (41.6527, 30.1661)
  line L74 (41.6527, 30.1661) -> (40.1509, 30.1661)
  line L75 (40.1509, 30.1661) -> (40.1509, 29.3313)
  line L76 (40.1509, 29.3313) -> (41.5514, 29.3313)
  line L77 (41.5514, 29.3313) -> (41.5514, 28.9706)
  line L78 (41.5514, 28.9706) -> (40.1509, 28.9706)
  line L79 (40.1509, 28.9706) -> (40.1509, 27.8394)
  line L80 (40.1509, 27.8394) -> (41.6527, 27.8394)
  line L81 (41.6527, 27.8394) -> (41.6527, 27.4788)
  line L82 (41.6527, 27.4788) -> (39.7458, 27.4788)
  point P0 (30.9203, 0)
  point P1 (30.9203, 26.0864)
  constraints: 2 end point, 2 midpoint, 1 point on line, 1 vertical, 2 other
emboss "Emboss2" sketch "Sketch9" operation add depth 0.55 direction (0, 1, 0)
fillet "Fillet6" radius 1 4 edges at (-12.5, -77.5, 16.0864) (0, -77.5, 26.0864) (12.5, -77.5, 16.0864) (0, -77.5, 6.0864)
body "Solid1"
